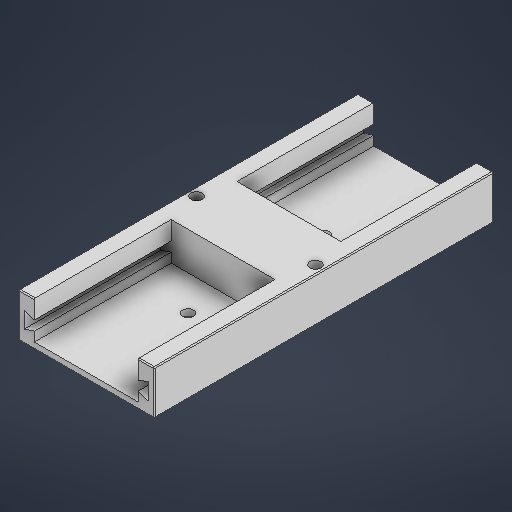
# Autodesk Inventor part: centralBodyThick
Saved by Autodesk Inventor 2026 (Build 300175000, 175)
## iProperties
Created: 2025-04-15
Part Number: centralBodyThick
Material: Generic
Document SubType Name: Modeling
Designer: Elizabeth
Density: 1 g/cm^3
Appearance: Default
Author: Elizabeth
Autodesk Inventor part; units mm, degrees
ref_plane "YZ Plane" through (0, 0, 0) normal (1, 0, 0) x (0, 1, 0)
ref_plane "XZ Plane" through (0, 0, 0) normal (0, 1, 0) x (-1, 0, 0)
ref_plane "XY Plane" through (0, 0, 0) normal (0, 0, 1) x (1, 0, 0)
sketch "Sketch1" plane through (0, 0, 0) normal (0, 0, 1) x (1, 0, 0)
  line L0 (0, 0) -> (40, 0)
  line L1 (40, 0) -> (40, 13)
  line L2 (40, 13) -> (0, 13)
  line L3 (0, 13) -> (0, 0)
  dimension "d0" = 40
  dimension "d1" = 13
  constraints: 8 end point, 2 parallel, 1 horizontal, 1 perpendicular
  measures "d0" distance of L2.end L1.end
  measures "d1" distance of L1.end L0.end
extrude "Extrusion1" add sketch "Sketch1" against normal blind 100
sketch "Sketch2" plane through (0, 0, 0) normal (0, 0, 1) x (1, 0, 0)
  line L0 (4.7, 1.898) -> (35.3, 1.898)
  line L1 (38.3, 8.5152) -> (38.3, 3.6828)
  line L2 (1.7, 8.5152) -> (1.7, 3.6828)
  line L3 (35.3, 7.5152) -> (38.3, 8.5152)
  line L4 (35.3, 7.5152) -> (35.3, 13)
  line L5 (35.3, 1.898) -> (35.3, 4.6828)
  line L6 (38.3, 3.6828) -> (35.3, 4.6828)
  line L7 (4.7, 7.5152) -> (1.7, 8.5152)
  line L8 (4.7, 13) -> (4.7, 7.5152)
  line L9 (4.7, 4.6828) -> (4.7, 1.898)
  line L10 (1.7, 3.6828) -> (4.7, 4.6828)
  line L11 (4.7, 13) -> (35.3, 13)
  point P0 (0, 13)
  point P1 (40, 13)
  constraints: 24 end point, 4 parallel, 2 point on line
extrude "Extrusion2" cut sketch "Sketch2" against normal blind 40.3
sketch "Sketch3" plane through (0, 0, -100) normal (0, 0, -1) x (-1, 0, 0)
  line L0 (-35.3, 1.898) -> (-4.7, 1.898)
  line L1 (-1.7, 8.5152) -> (-1.7, 3.6828)
  line L2 (-38.3, 8.5152) -> (-38.3, 3.6828)
  line L3 (-4.7, 7.5152) -> (-1.7, 8.5152)
  line L4 (-4.7, 7.5152) -> (-4.7, 13)
  line L5 (-4.7, 1.898) -> (-4.7, 4.6828)
  line L6 (-1.7, 3.6828) -> (-4.7, 4.6828)
  line L7 (-35.3, 7.5152) -> (-38.3, 8.5152)
  line L8 (-35.3, 13) -> (-35.3, 7.5152)
  line L9 (-35.3, 4.6828) -> (-35.3, 1.898)
  line L10 (-38.3, 3.6828) -> (-35.3, 4.6828)
  line L11 (-35.3, 13) -> (-4.7, 13)
  point P0 (-40, 13)
  point P1 (0, 13)
  constraints: 24 end point, 4 parallel, 2 point on line
extrude "Extrusion3" cut sketch "Sketch3" against normal blind 40.3
sketch "Sketch5" plane through (4.7, 1.898, 0) normal (0, 1, 0) x (1, 0, 0)
  circle A0 centre (15.3, 30) radius 1.65
  line L0 (35.3, 0) -> (35.3, 100) projected
  circle A1 centre (15.3, 70) radius 1.65
  point P0 (-4.7, 0)
  constraints: 2 centre point
extrude "Extrusion5" cut sketch "Sketch5" against normal blind 5
fillet "Fillet1" radius 0.3 14 edges at (2.35, 13, -100) (37.65, 13, -100) (0, 6.5, -100) (0, 13, -50) (0, 0, -50) (20, 0, -100) (40, 6.5, -100) (0, 6.5, 0) (40, 13, -50) (40, 0, -50) (20, 0, 0) (40, 6.5, 0) (2.35, 13, 0) (37.65, 13, 0)
sketch "Sketch6" plane through (4.7, 13, -40.3) normal (0, 1, 0) x (1, 0, 0)
  line L0 (-4.4, -40) -> (-4.4, 59.4) projected
  line L1 (-4.7, 59.4) -> (-4.7, -40) projected
  line L2 (35.3, -40) -> (35.3, 59.4) projected
  circle A0 centre (32.8, 9.7) radius 1.65
  circle A1 centre (-2.2, 9.7) radius 1.65
  point P0 (-4.7, -40.3)
  dimension "d29" = 3.3
  dimension "d30" = 3.3
  constraints: 2 centre point
  measures "d29" diameter of A0
  measures "d30" diameter of A1
extrude "Extrusion6" cut sketch "Sketch6" against normal blind 10
body "Solid1"
